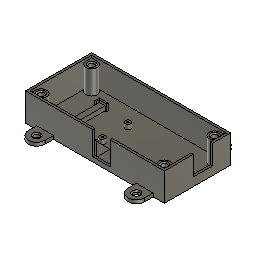
Thermux ESP32-POE-ISO Case (Autodesk Fusion 360 archive; units mm, degrees)
design "Base"
part number: 2026-08-16-18-28-22-034
Autodesk Fusion 360 part; units mm, degrees
sketch "Sketch1" plane through (0, 0, 0) normal (0, 0, 1) x (1, 0, 0)
  line L0 (-60, 27.5) -> (60, 27.5)
  line L1 (60, 27.5) -> (60, -27.5)
  line L2 (60, -27.5) -> (-60, -27.5)
  line L3 (-60, -27.5) -> (-60, 27.5)
  line L4 (-60, 27.5) -> (60, -27.5) construction
  line L5 (60, 27.5) -> (-60, -27.5) construction
  line L6 (62, -29.5) -> (-62, -29.5)
  line L7 (-62, -29.5) -> (-62, 29.5)
  line L8 (-62, 29.5) -> (62, 29.5)
  line L9 (62, 29.5) -> (62, -29.5)
  line L10 (-52, 29.5) -> (-37, 29.5)
  line L11 (-37, 29.5) -> (-37, 44.5)
  line L12 (-37, 44.5) -> (-52, 44.5)
  line L13 (-52, 44.5) -> (-52, 29.5)
  line L14 (0, 29.5) -> (0, -29.5) construction
  line L15 (-62, 0) -> (62, 0) construction
  line L16 (52, 29.5) -> (37, 29.5)
  line L17 (37, 29.5) -> (37, 44.5)
  line L18 (52, 44.5) -> (52, 29.5)
  line L19 (37, 44.5) -> (52, 44.5)
  line L20 (-52, -29.5) -> (-37, -29.5)
  line L21 (-37, -29.5) -> (-37, -44.5)
  line L22 (-52, -44.5) -> (-52, -29.5)
  line L23 (-37, -44.5) -> (-52, -44.5)
  line L24 (52, -29.5) -> (37, -29.5)
  line L25 (37, -29.5) -> (37, -44.5)
  line L26 (52, -44.5) -> (52, -29.5)
  line L27 (37, -44.5) -> (52, -44.5)
  line L28 (13.5, 29.5) -> (13.5, -29.5) construction
  line L29 (-2, -27.5) -> (13.5, -27.5)
  line L30 (13.5, -27.5) -> (13.5, -29.5)
  line L31 (13.5, -29.5) -> (-2, -29.5)
  line L32 (-2, -29.5) -> (-2, -27.5)
  line L33 (60, -3.5) -> (62, -3.5)
  line L34 (62, -3.5) -> (62, 13.5)
  line L35 (62, 13.5) -> (60, 13.5)
  line L36 (60, 13.5) -> (60, -3.5)
  line L37 (60, -7) -> (13.5, -7) construction
  line L38 (57, 0) -> (57, -27.5) construction
  circle A0 centre (57, -7) radius 2.5
  circle A1 centre (57, -7) radius 0.875
  line L39 (-62, -12) -> (0, -12) construction
  line L40 (-11, -27.5) -> (-11, 27.5) construction
  circle A2 centre (-11, -12) radius 2.5
  circle A3 centre (-11, -12) radius 0.875
  line L41 (-60, 11) -> (0, 11) construction
  circle A4 centre (-11, 11) radius 2.5
  circle A5 centre (-11, 11) radius 0.875
  line L42 (62, 13.5) -> (-60, 13.5) construction
  circle A6 centre (-44.5, 37) radius 7.5
  circle A7 centre (-44.5, 37) radius 2.5
  circle A8 centre (44.5, 37) radius 2.5
  circle A9 centre (-44.5, -37) radius 2.5
  circle A10 centre (44.5, -37) radius 2.5
  line L43 (-39, 27.5) -> (-39, -27.5) construction
  line L44 (-39, 13.5) -> (-34, 13.5)
  line L45 (-34, 13.5) -> (-34, -14.5)
  line L46 (-34, -14.5) -> (-39, -14.5)
  line L47 (-39, -14.5) -> (-39, 13.5)
  line L48 (-32.5, -16) -> (-40.5, -16)
  line L49 (-40.5, -16) -> (-40.5, 15)
  line L50 (-40.5, 15) -> (-32.5, 15)
  line L51 (-32.5, 15) -> (-32.5, -16)
  line L52 (-40.5, 11) -> (-39, 11)
  line L53 (-40.5, -12) -> (-39, -12)
  line L54 (-34, -14.5) -> (-32.5, -14.5)
  line L55 (-34, 13.5) -> (-32.5, 13.5)
  line L56 (-32.5, -0.5) -> (-11, -0.5) construction
  circle A11 centre (55, 22.5) radius 5
  circle A12 centre (55, 22.5) radius 2.5
  circle A13 centre (-55, 22.5) radius 2.5
  circle A14 centre (-55, 22.5) radius 5
  circle A15 centre (-55, -22.5) radius 5
  circle A16 centre (-55, -22.5) radius 2.5
  circle A17 centre (55, -22.5) radius 5
  circle A18 centre (55, -22.5) radius 2.5
  circle A19 centre (44.5, 37) radius 7.5
  circle A20 centre (-44.5, -37) radius 7.5
  circle A21 centre (44.5, -37) radius 7.5
  line L57 (-2, -27.5) -> (-4, -27.5)
  line L58 (-4, -27.5) -> (-4, -17.5)
  line L59 (-4, -17.5) -> (-2, -17.5)
  line L60 (-2, -17.5) -> (-2, -27.5)
  line L61 (-2, -27.5) -> (-7, -27.5)
  line L62 (-7, -27.5) -> (-7, -26)
  line L63 (-7, -26) -> (-2, -26)
  line L64 (-2, -26) -> (-2, -27.5)
  line L65 (-2, -26) -> (-4, -26)
  line L66 (-4, -26) -> (-4, -24)
  line L67 (-4, -24) -> (-2, -24)
  line L68 (-2, -24) -> (-2, -26)
  line L69 (5.75, -27.5) -> (5.75, -15.1319) construction
  line L70 (13.5, -27.5) -> (15.5, -27.5)
  line L71 (15.5, -27.5) -> (15.5, -17.5)
  line L72 (13.5, -17.5) -> (13.5, -27.5)
  line L73 (15.5, -17.5) -> (13.5, -17.5)
  line L74 (15.5, -24) -> (13.5, -24)
  line L75 (13.5, -26) -> (15.5, -26)
  circle A22 centre (-55, 22.5) radius 1.75
  circle A23 centre (55, 22.5) radius 1.75
  circle A24 centre (-55, -22.5) radius 1.75
  circle A25 centre (55, -22.5) radius 1.75
  dimension "d1" = 55
  dimension "d2" = 120
  dimension "d3" = -2
  dimension "d4" = 15
  dimension "d5" = 15
  dimension "d6" = 10
  dimension "d7" = 46.5
  dimension "d8" = 15.5
  dimension "d9" = 17
  dimension "d11" = 3
  dimension "d12" = 3.5
  dimension "d13" = 5
  dimension "d14" = 1.75
  dimension "d15" = 68
  dimension "d17" = 1.75
  dimension "d18" = 5
  dimension "d19" = 1.75
  dimension "d20" = 5
  dimension "d21" = 23
  dimension "d22" = 24
  dimension "d23" = 5
  dimension "d24" = 20.5
  dimension "d25" = 5
  dimension "d36" = 99
  dimension "d40" = 5
  dimension "d51" = 28
  dimension "d52" = 10
  dimension "d53" = 5
  dimension "d58" = 2
  dimension "d59" = 10
  dimension "d60" = 1.5
  dimension "d61" = 2
  dimension "d74" = 3.5
  dimension "d75" = 3.5
  dimension "d76" = 3.5
  dimension "d77" = 3.5
  constraint horizontal L0
  constraint perpendicular L0 L1
  constraint parallel L0 L2
  constraint parallel L1 L3
  constraint coincident L4 origin
  constraint coincident L5 origin
  constraint horizontal L10
  constraint vertical L11
  constraint horizontal L12
  constraint vertical L13
  constraint coincident L8 L10.start
  constraint midpoint L8 L14.start
  constraint midpoint L6 L14.end
  constraint midpoint L7 L15.start
  constraint midpoint L9 L15.end
  constraint symmetric L10.start L14 L16.start
  constraint symmetric L10.end L14 L16.end
  constraint symmetric L11.end L14 L17.end
  constraint symmetric L12.end L14 L18.start
  constraint symmetric L10.start L15 L20.start
  constraint symmetric L10.end L15 L20.end
  constraint symmetric L11.end L15 L21.end
  constraint symmetric L12.end L15 L22.start
  constraint symmetric L15 L16.start L24.start
  constraint symmetric L15 L16.end L24.end
  constraint symmetric L15 L17.end L25.end
  constraint symmetric L15 L18.start L26.start
  constraint coincident L8 L28.start
  constraint coincident L6 L28.end
  constraint vertical L28
  constraint horizontal L29
  constraint vertical L30
  constraint horizontal L31
  constraint vertical L32
  constraint coincident L2 L29.start
  constraint collinear L28 L30
  constraint horizontal L33
  constraint vertical L34
  constraint horizontal L35
  constraint vertical L36
  constraint coincident L9 L34.end
  constraint coincident L1 L33.start
  constraint coincident L1 L37.start
  constraint coincident L28 L37.end
  constraint coincident L15 L38.start
  constraint coincident L2 L38.end
  constraint vertical L38
  constraint horizontal L37
  constraint coincident L37 A0.centre
  constraint coincident L38 A0.centre
  constraint concentric A0 A1
  constraint coincident L7 L39.start
  constraint coincident L14 L39.end
  constraint coincident L2 L40.start
  constraint coincident L0 L40.end
  constraint vertical L40
  constraint horizontal L39
  constraint coincident L39 A2.centre
  constraint coincident L40 A2.centre
  constraint concentric A2 A3
  constraint coincident L3 L41.start
  constraint coincident L14 L41.end
  constraint horizontal L41
  constraint coincident L41 A4.centre
  constraint coincident L40 A4.centre
  constraint concentric A4 A5
  constraint coincident L3 L42.end
  constraint horizontal L42
  constraint tangent L11 A6
  constraint tangent L13 A6
  constraint tangent L12 A6
  constraint concentric A6 A7
  constraint symmetric L14 A7 A8
  constraint symmetric L15 A7 A9
  constraint symmetric L15 A8 A10
  constraint coincident L0 L43.start
  constraint coincident L2 L43.end
  constraint vertical L43
  constraint horizontal L44
  constraint vertical L45
  constraint horizontal L46
  constraint vertical L47
  constraint coincident L43 L44.start
  constraint coincident L49 L52.start
  constraint coincident L41 L52.start
  constraint coincident L43 L52.end
  constraint coincident L39 L53.start
  constraint coincident L49 L53.start
  constraint coincident L43 L53.end
  constraint horizontal L52
  constraint horizontal L53
  constraint coincident L51 L54.end
  constraint coincident L51 L55.end
  constraint horizontal L55
  constraint horizontal L54
  constraint coincident L47.start L46
  constraint coincident L46.end L47.start
  constraint collinear L42 L44
  constraint coincident L40 L56.end
  constraint horizontal L56
  constraint midpoint L51 L56.start
  constraint concentric A11 A12
  constraint tangent L0 A11
  constraint tangent L1 A11
  constraint symmetric L14 A11 A14
  constraint symmetric L14 A12 A13
  constraint symmetric L15 A11 A17
  constraint symmetric L15 A12 A18
  constraint symmetric L15 A13 A16
  constraint symmetric L15 A14 A15
  constraint symmetric L14 A6 A19
  constraint symmetric L15 A6 A20
  constraint symmetric L15 A19 A21
  constraint horizontal L57
  constraint vertical L58
  constraint horizontal L59
  constraint vertical L60
  constraint horizontal L61
  constraint vertical L62
  constraint horizontal L63
  constraint vertical L64
  constraint horizontal L65
  constraint vertical L66
  constraint horizontal L67
  constraint vertical L68
  constraint coincident L58 L66.end
  constraint midpoint L29 L69.start
  constraint vertical L69
  constraint symmetric L29.start L69 L29.end
  constraint symmetric L57.end L69 L70.end
  constraint symmetric L58.end L69 L71.end
  constraint symmetric L59.end L69 L72.start
  constraint symmetric L63.end L69 L75.start
  constraint symmetric L65.end L69 L75.end
  constraint symmetric L66.end L69 L74.start
  constraint symmetric L67.end L69 L74.end
  constraint concentric A13 A22
  constraint concentric A11 A23
  constraint concentric A16 A24
  constraint concentric A17 A25
  measures "d1" distance of L0.start L2.end
  measures "d2" distance of L0.start L0.end
  measures "d4" distance of L11.end L12.end
  measures "d5" distance of L10.end L11.end
  measures "d6" distance of L7 L13
  measures "d7" distance of L1 L28
  measures "d8" distance of L30 L32
  measures "d9" distance of L33 L35
  measures "d11" distance of L1 L38
  measures "d12" distance of L33 L37
  measures "d13" diameter of A0
  measures "d14" diameter of A1
  measures "d15" distance of L38 L40
  measures "d17" diameter of A3
  measures "d18" diameter of A2
  measures "d19" diameter of A5
  measures "d20" diameter of A4
  measures "d21" distance of L39 L41
  measures "d22" distance of L2 L33
  measures "d23" distance of L37 L39
  measures "d24" distance of L2 L37
  measures "d25" diameter of A7
  measures "d36" distance of L1 L43
  measures "d40" distance of L44.start L44.end
  measures "d51" distance of L44 L46
  measures "d52" diameter of A11
  measures "d53" diameter of A12
  measures "d58" distance of L29.start L57.end
  measures "d59" distance of L29.start L59.end
  measures "d60" distance of L29.start L63.end
  measures "d61" distance of L63 L67
  measures "d74" diameter of A22
  measures "d75" diameter of A23
  measures "d76" diameter of A24
  measures "d77" diameter of A25
extrude "Extrude1" add sketch "Sketch1" against normal blind 2 contours L0 L1 L2 L3 L6 L7 L8 L9 L10 L16 L20 L32 L35 L57 L61 | L0 L3 A14 | L0 L1 L2 L3 L29 L36 A11 A14 A15 A17 L58 L59 L60 L62 L63 L64 L66 L68 L71 L72 L73 | A14 | L0 L1 A11 | A11 | L2 L3 A15 | A15 | L1 L9 L33 L34 L35 L36 | L2 L58 L61 L62 L63 | L1 L2 L6 L9 L24 L30 L33 L70 | L2 L57 L58 L60 L61 L63 L64 L65 | A17 | L1 L2 A17 | L2 L6 L29 L30 L31 L32 | L58 L60 L63 L65 L66 L67 L68 | L2 L70 L71 L72 L75 | L58 L59 L60 L67 | L71 L72 L74 L75 | L71 L72 L73 L74 | A0 | A1 | A2 | A3 | A4 | A5 | L44 L47 L49 L50 L51 L52 L55 | L44 L45 L46 L47 | L45 L51 L54 L55 | L47 L49 L52 L53 | L46 L47 L48 L49 L51 L53 L54 | A12 | A13 | A16 | A18 | A22 | A23 | A24 | A25 makes body 1
extrude "Extrude2" add sketch "Sketch1" along normal blind 23 contours L0 L1 L2 L3 L6 L7 L8 L9 L10 L16 L20 L32 L35 L57 L61 | L1 L2 L6 L9 L24 L30 L33 L70 bodies 1
extrude "Extrude3" add sketch "Sketch1" along normal blind 4 contours A0 | A2 | A4 bodies 1
extrude "Extrude5" add sketch "Sketch1" along normal up to surface (4 mm away) separate body contours L44 L45 L46 L47 makes body 2
extrude "Extrude6" add sketch "Sketch1" along normal up to surface (6 mm away) contours L44 L47 L49 L50 L51 L52 L55 | L46 L47 L48 L49 L51 L53 L54 bodies 1 2
extrude "Extrude7" add sketch "Sketch1" along normal up to surface (5.5 mm away) contours L1 L9 L33 L34 L35 L36 bodies 1
extrude "Extrude8" add sketch "Sketch1" along normal blind 2 contours L2 L6 L29 L30 L31 L32 bodies 1
extrude "Extrude9" add sketch "Sketch1" along normal up to surface (21 mm away) contours L0 L3 A14 | A14 | L0 L1 A11 | A11 | L2 L3 A15 | A15 | A17 | L1 L2 A17 bodies 1
extrude "Extrude10" add sketch "Sketch1" along normal up to surface (16.5 mm away) contours A12 | A13 | A16 | A18 | A22 | A23 | A24 | A25 bodies 1
extrude "Extrude11" add sketch "Sketch1" along normal up to surface (12 mm away) contours L58 L60 L63 L65 L66 L67 L68 | L71 L72 L74 L75 bodies 1
chamfer "Chamfer1" distance 10 angle 45 2 edges at (14.5, -24, 0) (-3, -24, 0) tangent chain off on bodies 1
extrude "Extrude12" add sketch "Sketch1" along normal blind 1 and the other way up to surface (2 mm away) contours L8 L16 L18 A19 | L6 L24 L26 A21 | L8 L16 L17 A19 | A19 | L6 L20 L21 A20 | L6 L24 L25 A21 | A21 | L6 L20 L22 A20 | A20 | L8 L10 L11 A6 | L8 L10 L13 A6 | A6 bodies 1
chamfer "Chamfer2" distance 1 angle 45 4 edges at (-46.8308, -36.096, 1) (42.1692, -36.096, 1) (42.1692, 37.904, 1) (-46.8308, 37.904, 1) tangent chain off on bodies 1
chamfer "Chamfer3" distance 1 angle 45 4 edges at (-57.3308, 21.596, 21) (-57.3308, -23.404, 21) (52.6692, -23.404, 21) (52.6692, 21.596, 21) tangent chain off on bodies 1
extrude "Extrude13" cut sketch "Sketch1" against normal blind 5 from surface at 16.5 contours A22 | A23 | A24 | A25 bodies 1
